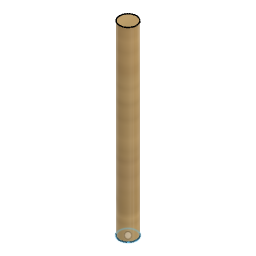
_Pin.3e5627a4-a375-4992-b748-745666143fb8 (Autodesk Fusion 360 design; units mm, degrees)
Autodesk Fusion 360 part; units mm, degrees
sketch "sketch 268" plane through (0, 0, 0) normal (0, 0, 1) x (1, 0, 0)
  circle A0 centre (-3.1462, 63.4493) radius 6.35
extrude "Extrude1" add sketch "sketch 268" along normal blind 139.7
